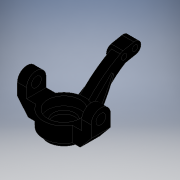
# Autodesk Inventor part: RCT-P006_steering_knuckle
Saved by Autodesk Inventor 2018.1 (Build 221171000, 171)
## iProperties
Created: 2018-12-11
Part Number: RCT-P006_steering_knuckle
Material: Generic
Document SubType Name: Modeling
Designer: Ehecatl Eli
Density: 1 g/cm^3
Appearance: Default
Author: Ehecatl Eli
Autodesk Inventor part; units mm, degrees
ref_plane "YZ Plane" through (0, 0, 0) normal (1, 0, 0) x (0, 1, 0)
ref_plane "XZ Plane" through (0, 0, 0) normal (0, 1, 0) x (-1, 0, 0)
ref_plane "XY Plane" through (0, 0, 0) normal (0, 0, 1) x (1, 0, 0)
sketch "Sketch1" plane through (0, 0, 0) normal (0, 0, 1) x (1, 0, 0)
  line L0 (17, 4.5) -> (17, -4.5)
  line L1 (-17, -4.5) -> (-17, 4.5)
  arc A0 (-8.3666, -4.5) -> (8.3666, -4.5) centre (0, 0) ccw
  arc A1 (8.3666, 4.5) -> (-8.3666, 4.5) centre (0, 0) ccw
  line L2 (-17, 4.5) -> (-8.3666, 4.5)
  line L3 (8.3666, 4.5) -> (17, 4.5)
  line L4 (17, -4.5) -> (8.3666, -4.5)
  line L5 (-8.3666, -4.5) -> (-17, -4.5)
  line L6 (-17, 4.5) -> (17, -4.5) construction
  line L7 (-17, -4.5) -> (17, 4.5) construction
  point P0 (0, 0)
  point P1 (0, 0)
  dimension "d0" = 9
  dimension "d1" = 34
  dimension "d2" = 9.5
  dimension "d3" = 9
  dimension "d4" = 9.5
  dimension "d12" = 4.5
  constraints: 16 end point, 5 parallel, 4 point on circle, 2 centre point, 2 coincident, 2 horizontal, 2 midpoint, 2 perpendicular
  measures "d0" distance of L1.start L1.end
  measures "d1" distance between parallel lines of L0 L1
  measures "d2" radius of A1
  measures "d3" distance of L0.start L0.end
  measures "d4" radius of A0
  measures "d12" distance from line of point (0, 0) L5
extrude "Extrusion1" add sketch "Sketch1" along normal blind 7
sketch "Sketch2" plane through (17, -4.5, 0) normal (1, 0, 0) x (0, 0, -1)
  arc A0 (-11.5, 9) -> (-11.5, 0) centre (-11.5, 4.5) ccw
  circle A1 centre (-11.5, 4.5) radius 2.25
  line L0 (-7, 9) -> (-11.5, 9)
  line L1 (-11.5, 0) -> (-7, 0)
  line L2 (-7, 0) -> (-7, 9)
  point P0 (0, 4.5)
  point P1 (-7, 0)
  dimension "d7" = 9
  dimension "d8" = 4.5
  dimension "d9" = 9
  constraints: 6 end point, 2 centre point, 2 coincident, 2 horizontal, 2 point on circle, 2 tangent, 1 parallel, 1 vertical
  measures "d7" diameter of A0
  measures "d8" diameter of A1
extrude "Extrusion2" add sketch "Sketch2" against normal blind 4.3
extrude "Extrusion3" add sketch "Sketch2" along normal blind 4.3 from surface at -34
sketch "Sketch3" plane through (-17, -4.5, 0) normal (0, -1, 0) x (1, 0, 0)
  line L0 (0, 6) -> (0, 0)
  line L1 (0, 0) -> (5, 0)
  line L2 (5, 0) -> (0, 6)
  line L3 (29, 0) -> (34, 0)
  line L4 (34, 0) -> (34, 6)
  line L5 (34, 6) -> (29, 0)
  point P0 (17, 0)
  dimension "d15" = 6
  dimension "d16" = 5
  dimension "d17" = 6
  dimension "d18" = 5
  constraints: 12 end point, 2 coincident, 2 perpendicular, 1 horizontal, 1 vertical
  measures "d15" distance of L0.start L0.end
  measures "d16" distance of L0.end L1.end
  measures "d17" distance of L3.end L4.end
  measures "d18" distance of L3.start L3.end
extrude "Extrusion4" cut sketch "Sketch3" against normal up to next
sketch "Sketch4" plane through (0, 0, 0) normal (0, 0, -1) x (-1, 0, 0)
  circle A0 centre (0, 0) radius 7.5
  dimension "d21" = 15
  constraints: 1 centre point, 1 coincident
  measures "d21" diameter of A0
extrude "Extrusion5" add sketch "Sketch4" along normal blind 2.5
sketch "Sketch5" plane through (0, 0, 7) normal (0, 0, 1) x (1, 0, 0)
  circle A0 centre (0, 0) radius 7.5
  dimension "d24" = 15
  constraints: 1 centre point, 1 coincident
  measures "d24" diameter of A0
extrude "Extrusion6" cut sketch "Sketch5" against normal blind 4
sketch "Sketch6" plane through (0, 0, -2.5) normal (0, 0, -1) x (-1, 0, 0)
  circle A0 centre (0, 0) radius 5.5
  dimension "d27" = 11
  constraints: 1 centre point, 1 coincident
  measures "d27" diameter of A0
extrude "Extrusion7" cut sketch "Sketch6" against normal blind 4
sketch "Sketch7" plane through (0, 0, 1.5) normal (0, 0, -1) x (-1, 0, 0)
  circle A0 centre (0, 0) radius 5
  dimension "d30" = 10
  constraints: 1 centre point, 1 coincident
  measures "d30" diameter of A0
extrude "Extrusion8" cut sketch "Sketch7" against normal up to next
sketch "Sketch9" plane through (0, 0, 0) normal (1, 0, 0) x (0, 1, 0)
  arc A0 (31.2893, 14.3034) -> (30.2107, 19.6966) centre (30.75, 17) ccw
  line L0 (-9.5504, 0) -> (57.3026, 0) projected
  line L1 (0, -37.6235) -> (0, 29.8791) projected
  circle A1 centre (30.75, 17) radius 1.25
  arc A2 (25.2107, 18.6966) -> (23.9154, 18.0486) centre (25.75, 16) ccw
  circle A3 centre (25.75, 16) radius 1.25
  line L2 (9.5, 7) -> (9.5, 0)
  line L3 (9.5, 0) -> (12.3425, 0)
  line L4 (25.2107, 18.6966) -> (30.2107, 19.6966)
  line L5 (26.2893, 13.3034) -> (31.2893, 14.3034)
  arc A4 (23.9154, 18.0486) -> (9.5, 7) centre (47.7522, -27.9802) ccw
  arc A5 (26.2893, 13.3034) -> (14.061, 0.9769) centre (44.8843, -17.3723) ccw
  arc A6 (12.3425, 0) -> (14.061, 0.9769) centre (12.3425, 2) ccw
  line L6 (8.5, 7) -> (9.5, 7)
  line L7 (9.5, 7) -> (9.5, 0)
  line L8 (9.5, 0) -> (8.5, 0)
  line L9 (8.5, 0) -> (8.5, 7)
  point P0 (0, 0)
  point P1 (13.5, 0)
  dimension "d53" = 5.5
  dimension "d54" = 17
  dimension "d55" = 30.75
  dimension "d56" = 2.5
  dimension "d57" = 16
  dimension "d58" = 25.75
  dimension "d59" = 4
  dimension "d60" = 7
  dimension "d61" = 9.5
  dimension "d62" = 0
  dimension "d63" = 51.8348
  dimension "d64" = 35.8716
  dimension "d65" = 2
  dimension "d88" = 7
  dimension "d89" = 1
  dimension "d90" = 0
  dimension "d91" = 0
  constraints: 16 end point, 11 point on circle, 7 centre point, 6 tangent, 2 coincident, 2 equal radius, 2 parallel, 2 perpendicular, 1 horizontal, 1 point on line, 1 vertical
  measures "d53" diameter of A0
  measures "d54" distance from line of L0 A0.centre
  measures "d55" distance from line of L1 A0.centre
  measures "d56" diameter of A1
  measures "d57" distance from line of L0 A2.centre
  measures "d58" distance from line of L1 A2.centre
  measures "d59" distance of L2.end point (13.5, 0)
  measures "d60" distance of L2.start L2.end
  measures "d61" distance between parallel lines of L1 L2
  measures "d62" distance between parallel lines of L0 L3
  measures "d63" radius of A4
  measures "d64" radius of A5
  measures "d65" radius of A6
  measures "d88" distance of L8.end L6.start
  measures "d89" distance of L7.end L8.end
  measures "d90" distance between parallel lines of L2 L7
  measures "d91" distance between parallel lines of L0 L8
extrude "Extrusion9" add sketch "Sketch9" along normal mid plane 4 contours L5 A5 A6 L0 L2 A4 A2 L4 A0
sketch "Sketch10" plane through (0, 0, 0) normal (1, 0, 0) x (0, 1, 0)
  arc A0 (25.2107, 18.6966) -> (26.2893, 13.3034) centre (25.75, 16) ccw
  circle A1 centre (25.75, 16) radius 1.25 projected
  arc A2 (31.2893, 14.3034) -> (30.2107, 19.6966) centre (30.75, 17) ccw
  circle A3 centre (25.75, 16) radius 1.25
  circle A4 centre (30.75, 17) radius 1.25
  circle A5 centre (30.75, 17) radius 1.25 projected
  line L0 (25.2107, 18.6966) -> (30.2107, 19.6966)
  line L1 (26.2893, 13.3034) -> (31.2893, 14.3034)
  point P0 (0, 0)
  dimension "d68" = 5.5
  dimension "d69" = 2.5
  constraints: 4 centre point, 4 end point, 4 point on circle, 4 tangent, 2 coincident, 2 concentric, 2 equal radius
  measures "d68" diameter of A0
  measures "d69" diameter of A3
extrude "Extrusion10" add sketch "Sketch10" against normal blind 3.5
sketch "Sketch11" plane through (0, 0, 0) normal (1, 0, 0) x (0, 1, 0)
  line L0 (-4.2102, 0) -> (25.2612, 0) projected
  line L1 (0, -2.5102) -> (0, 15.0612) projected
  line L2 (19.9196, 12.551) -> (11.6686, 4.3)
  line L3 (11.6686, 4.3) -> (0, 4.3)
  line L4 (21.051, 11.4196) -> (12.3314, 2.7)
  line L5 (12.3314, 2.7) -> (0, 2.7)
  line L6 (21.051, 11.4196) -> (19.9196, 12.551)
  line L7 (0, 4.3) -> (0, 2.7)
  point P0 (0, 0)
  constraints: 12 end point, 2 perpendicular, 2 point on line
extrude "Extrusion11" add sketch "Sketch11" along normal mid plane 12
extrude "Extrusion12" cut sketch "Sketch5" against normal blind 4
extrude "Extrusion13" cut sketch "Sketch7" against normal through all
sketch "Sketch12" plane through (0, 0, 0) normal (0, 0, 1) x (1, 0, 0)
  line L0 (6, 7.3655) -> (6, 12.3314) projected
  line L1 (2, 21.051) -> (6, 21.051) projected
  arc A0 (6, 7.3655) -> (2, 21.051) centre (-49.0316, -1.2919) ccw
  line L2 (0, 0) -> (0, 16.5543) construction
  arc A1 (-2, 21.051) -> (-6, 7.3655) centre (49.0316, -1.2919) ccw
  line L3 (2, 26.2893) -> (2, 14.061) construction
  line L4 (2, 21.051) -> (6, 21.051)
  line L5 (6, 7.3655) -> (6, 21.051)
  line L6 (-6, 7.3655) -> (-6, 21.051)
  line L7 (-2, 21.051) -> (-6, 21.051)
  constraints: 10 end point, 4 point on circle, 3 symmetric about line, 2 centre point, 2 perpendicular, 2 vertical, 1 coincident, 1 point on line, 1 other
extrude "Extrusion14" cut sketch "Sketch12" along normal up to next
sketch "Sketch13" plane through (0, 0, 0) normal (1, 0, 0) x (0, 1, 0)
  line L0 (8.5, 7) -> (9.5, 7)
  line L1 (9.5, 7) -> (9.5, 0)
  line L2 (9.5, 0) -> (8.5, 0)
  line L3 (8.5, 0) -> (8.5, 7)
  line L4 (0, -6.95) -> (0, 24.2) projected
  line L5 (-18.1, 0) -> (42.1, 0) projected
  point P0 (0, 0)
  dimension "d92" = 7
  dimension "d93" = 1
  dimension "d94" = 9.5
  dimension "d95" = 0
  constraints: 8 end point, 2 parallel, 1 horizontal, 1 perpendicular
  measures "d92" distance of L0.end L1.end
  measures "d93" distance of L0.start L0.end
  measures "d94" distance between parallel lines of L4 L1
  measures "d95" distance between parallel lines of L5 L2
extrude "Extrusion15" add sketch "Sketch13" along normal mid plane 4
body "Solid1"
